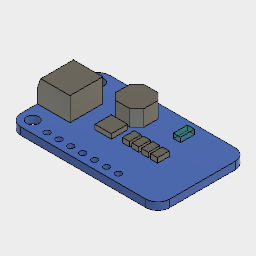
2190 Verter 5V USB (Autodesk Fusion 360 design; units mm, degrees)
Autodesk Fusion 360 part; units mm, degrees
sketch "Sketch1" plane through (0, 0, 0) normal (0, 0, 1) x (1, 0, 0)
  line L0 (0, 0) -> (31.75, 0)
  line L1 (31.75, 0) -> (31.75, 19.05)
  line L2 (31.75, 19.05) -> (0, 19.05)
  line L3 (0, 19.05) -> (0, 0)
  circle A0 centre (2.54, 2.54) radius 1.27
  circle A1 centre (2.54, 16.51) radius 1.27
  line L4 (7, 6.025) -> (0, 6.025)
  line L5 (0, 6.025) -> (0, 13.025)
  line L6 (0, 13.025) -> (7, 13.025)
  line L7 (7, 13.025) -> (7, 6.025)
  line L8 (7, 6.025) -> (0, 13.025) construction
  line L9 (0, 6.025) -> (7, 13.025) construction
  circle A2 centre (3.4993, 10.795) radius 0.635
  circle A3 centre (3.5007, 8.255) radius 0.635
  line L10 (3.4993, 10.795) -> (3.5007, 8.255) construction
  line L11 (15.7, 11.605) -> (9.7, 11.605)
  line L12 (9.7, 11.605) -> (9.7, 17.605)
  line L13 (9.7, 17.605) -> (15.7, 17.605)
  line L14 (15.7, 17.605) -> (15.7, 11.605)
  line L15 (15.7, 11.605) -> (9.7, 17.605) construction
  line L16 (9.7, 11.605) -> (15.7, 17.605) construction
  line L17 (14.45, 7.394) -> (10.95, 7.394)
  line L18 (10.95, 7.394) -> (10.95, 10.894)
  line L19 (10.95, 10.894) -> (14.45, 10.894)
  line L20 (14.45, 10.894) -> (14.45, 7.394)
  line L21 (14.45, 7.394) -> (10.95, 10.894) construction
  line L22 (10.95, 7.394) -> (14.45, 10.894) construction
  line L23 (17.8162, 7.894) -> (16.3162, 7.894)
  line L24 (16.3162, 7.894) -> (16.3162, 10.394)
  line L25 (16.3162, 10.394) -> (17.8162, 10.394)
  line L26 (17.8162, 10.394) -> (17.8162, 7.894)
  line L27 (17.8162, 7.894) -> (16.3162, 10.394) construction
  line L28 (16.3162, 7.894) -> (17.8162, 10.394) construction
  line L29 (22.467, 14.121) -> (20.967, 14.121)
  line L30 (20.967, 14.121) -> (20.967, 17.121)
  line L31 (20.967, 17.121) -> (22.467, 17.121)
  line L32 (22.467, 17.121) -> (22.467, 14.121)
  line L33 (22.467, 14.121) -> (20.967, 17.121) construction
  line L34 (20.967, 14.121) -> (22.467, 17.121) construction
  circle A4 centre (13.97, 1.778) radius 0.635
  point P0 (3.5, 9.525)
  point P1 (12.7, 14.605)
  point P2 (12.7, 9.144)
  point P3 (17.0662, 9.144)
  point P4 (21.717, 15.621)
  dimension "d1" = 31.75
  dimension "d2" = 19.05
  dimension "d3" = 2.54
  dimension "d4" = 2.54
  dimension "d5" = 2.54
  dimension "d6" = 2.54
  dimension "d7" = 16.51
  dimension "d8" = 2.54
  dimension "d12" = 7
  dimension "d13" = 7
  dimension "d14" = 9.525
  dimension "d15" = 1.27
  dimension "d16" = 1.27
  dimension "d17" = 2.54
  dimension "d18" = 6
  dimension "d19" = 6
  dimension "d20" = 14.605
  dimension "d21" = 12.7
  dimension "d26" = 3.5
  dimension "d27" = 3.5
  dimension "d28" = 9.144
  dimension "d29" = 12.7
  dimension "d33" = 2.5
  dimension "d34" = 1.5
  dimension "d35" = 9.144
  dimension "d43" = 3
  dimension "d44" = 1.5
  dimension "d45" = 21.717
  dimension "d46" = 15.621
  dimension "d50" = 1.27
  dimension "d51" = 1.778
  dimension "d52" = 13.97
  measures "d1" distance of L1.end L2.end
  measures "d2" distance of L0.start L2.end
  measures "d3" diameter of A0
  measures "d4" distance of L3 A0.centre
  measures "d5" distance of L0 A0.centre
  measures "d6" diameter of A1
  measures "d7" distance of L0 A1.centre
  measures "d8" distance of L3 A1.centre
  measures "d12" distance of L4.end L5.end
  measures "d13" distance of L5.end L6.end
  measures "d14" distance of L0 P0
  measures "d15" diameter of A2
  measures "d16" diameter of A3
  measures "d17" distance of A2.centre A3.centre
  measures "d18" distance of L12.end L13.end
  measures "d19" distance of L11.end L12.end
  measures "d20" distance of L0 P1
  measures "d21" distance of L3 P1
  measures "d26" distance of L17.end L18.end
  measures "d27" distance of L18.end L19.end
  measures "d28" distance of L0 P2
  measures "d29" distance of L3 P2
  measures "d33" distance of L23.end L24.end
  measures "d34" distance of L24.end L25.end
  measures "d35" distance of L0 P3
  measures "d43" distance of L29.end L30.end
  measures "d44" distance of L30.end L31.end
  measures "d45" distance of L3 P4
  measures "d46" distance of L0 P4
  measures "d50" diameter of A4
  measures "d51" distance of L0 A4.centre
  measures "d52" distance of L3 A4.centre
extrude "Extrude1" add sketch "Sketch1" along normal blind 1.6 contours L0 L1 L2 L3 L4 L6 L7 | L3 L4 L5 L6 L7 | L11 L12 L13 L14 | L17 L18 L19 L20 | L23 L24 L25 L26 | L29 L30 L31 L32 | A4 makes body 1
fillet "Fillet1" radius 2.54 4 edges at (0, 0, 0.8) (0, 19.05, 0.8) (31.75, 19.05, 0.8) (31.75, 0, 0.8) on bodies 1
extrude "Extrude2" add sketch "Sketch1" along normal blind 3.4 from surface at 1.6 separate body contours L11 L12 L13 L14 makes body 2
chamfer "Chamfer1" distance 1.5 angle 45 4 edges at (9.7, 11.605, 3.3) (9.7, 17.605, 3.3) (15.7, 17.605, 3.3) (15.7, 11.605, 3.3) on bodies 2
extrude "Extrude3" add sketch "Sketch1" along normal blind 1 from surface at 1.6 separate body contours L17 L18 L19 L20 makes body 3
extrude "Extrude4" add sketch "Sketch1" along normal blind 1 from surface at 1.6 separate body contours L23 L24 L25 L26 makes body 4
pattern_linear "R-Pattern1" count 4 spacing 2 along (1, 0, 0) of "Extrude4" makes body 5 makes body 6 makes body 7
extrude "Extrude5" add sketch "Sketch1" along normal blind 1 from surface at 1.6 separate body contours L29 L30 L31 L32 makes body 8
extrude "Extrude6" cut sketch "Sketch1" along normal up to surface (1.6 mm away) contours A4 bodies 1
pattern_linear "R-Pattern2" count 4 spacing 2.54 along (1, 0, 0) of "Extrude6"
pattern_linear "R-Pattern3" count 4 spacing 2.54 along (-1, 0, 0) of "Extrude6"
extrude "Extrude7" add sketch "Sketch1" along normal blind 3 from surface at 1.6 separate body contours L3 L4 L5 L6 L7 | A2 | A3 makes body 9
sketch "Sketch2" plane through (0, 0, 4.6) normal (0, 0, 1) x (-1, 0, 0)
  line L0 (-7, -6.025) -> (-7, -13.025)
  line L1 (-7, -13.025) -> (0, -13.025)
  line L2 (0, -13.025) -> (0, -6.025)
  line L3 (0, -6.025) -> (-7, -6.025)
sketch "Sketch3" plane through (0, 0, 0) normal (0, 1, 0) x (1, 0, 0)
  line L0 (7, -4.6) -> (0, -4.6)
  line L1 (7, -4.6) -> (7, -6.6)
  line L2 (7, -6.6) -> (0.7347, -6.6)
  line L3 (0.7347, -6.6) -> (0, -4.6)
  point P0 (7, -4.6)
  dimension "d66" = 2
  measures "d66" distance of P0 L1.end
extrude "Extrude8" add sketch "Sketch3" along normal up to surface (7 mm away) from surface at 6.025 bodies 9
sketch "Sketch4" plane through (0, 0, 0) normal (-1, 0, 0) x (0, -1, 0)
  line L0 (-13.025, 1.6) -> (-6.025, 1.6)
  line L1 (-6.025, 1.6) -> (-6.025, 4.6)
  line L2 (-6.025, 4.6) -> (-13.025, 4.6)
  line L3 (-13.025, 4.6) -> (-13.025, 1.6)
  line L4 (-6.025, 3.1) -> (-13.025, 3.1) construction
  circle A0 centre (-11.025, 3.1) radius 0.75
  circle A1 centre (-8.025, 3.1) radius 0.75
  line L5 (-12.625, 4.2) -> (-6.425, 4.2)
  line L6 (-6.425, 4.2) -> (-6.425, 2)
  line L7 (-6.425, 2) -> (-12.625, 2)
  line L8 (-12.625, 2) -> (-12.625, 4.2)
  line L9 (-9.725, 4.2) -> (-9.325, 4.2)
  line L10 (-9.325, 4.2) -> (-9.325, 2)
  line L11 (-9.325, 2) -> (-9.725, 2)
  line L12 (-9.725, 2) -> (-9.725, 4.2)
  dimension "d70" = 1.5
  dimension "d71" = 1.5
  dimension "d72" = 3
  dimension "d73" = 2
  dimension "d76" = 0.4
  dimension "d77" = 0.4
  dimension "d78" = 0.4
  dimension "d79" = 0.4
  dimension "d82" = 0.4
  measures "d70" diameter of A0
  measures "d71" diameter of A1
  measures "d72" distance of A0.centre A1.centre
  measures "d73" distance of L4.end A0.centre
  measures "d76" distance of L1 L6
  measures "d77" distance of L2 L5
  measures "d78" distance of L0 L7
  measures "d79" distance of L3 L8
  measures "d82" distance of L9.start L9.end
extrude "Extrude9" cut sketch "Sketch4" against normal blind 2 contours A0 | A1 bodies 9
extrude "Extrude10" cut sketch "Sketch4" against normal blind 0.2 contours L5 L7 L8 L12 | L5 L6 L7 L10 bodies 9
